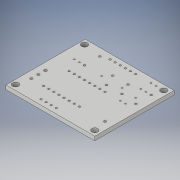
# Autodesk Inventor part: bard
Saved by Autodesk Inventor 2019 (Build 230136000, 136)
## iProperties
Created: 2020-01-03
Part Number: bard
Material: Типовые
Document SubType Name: Modeling
Designer: Петров Иван
Density: 1 g/cm^3
Appearance: По умолчанию
Author: Петров Иван
Autodesk Inventor part; units mm, degrees
ref_plane "YZ Plane" through (0, 0, 0) normal (1, 0, 0) x (0, 1, 0)
ref_plane "XZ Plane" through (0, 0, 0) normal (0, 1, 0) x (-1, 0, 0)
ref_plane "XY Plane" through (0, 0, 0) normal (0, 0, 1) x (1, 0, 0)
sketch "Эскиз1" plane through (0, 0, 0) normal (0, 1, 0) x (-1, 0, 0)
  arc A0 (18.669, 20.0698) -> (19.177, 20.0622) centre (18.923, 20.066) ccw
  arc A1 (19.304, 28.4442) -> (18.796, 28.4518) centre (19.05, 28.448) ccw
  line L0 (18.923, 20.066) -> (19.05, 28.448)
  arc A2 (32.004, 28.575) -> (31.496, 28.575) centre (31.75, 28.575) ccw
  line L1 (31.75, 28.575) -> (31.75, 21.209)
  arc A3 (31.496, 21.209) -> (32.004, 21.209) centre (31.75, 21.209) ccw
  arc A4 (34.163, 20.0622) -> (34.671, 20.0698) centre (34.417, 20.066) ccw
  arc A5 (34.544, 28.5788) -> (34.036, 28.5712) centre (34.29, 28.575) ccw
  line L2 (34.29, 28.575) -> (34.417, 20.066)
  line L3 (0, 0) -> (44.12, 0)
  line L4 (44.12, 0) -> (44.12, 39.36)
  line L5 (44.12, 39.36) -> (0, 39.36)
  line L6 (0, 39.36) -> (0, 0)
  circle A6 centre (2.54, 36.83) radius 1.5
  circle A7 centre (41.91, 36.83) radius 1.5
  circle A8 centre (41.91, 2.54) radius 1.5
  circle A9 centre (2.54, 2.54) radius 1.5
  line L7 (15.24, 5.588) -> (15.24, 0)
  arc A10 (16.51, 0.0318) -> (16.51, -0.0318) centre (16.51, 0) ccw
  line L8 (30.48, 5.588) -> (30.48, 0)
  arc A11 (30.4482, 0) -> (30.5118, 0) centre (30.48, 0) ccw
  arc A12 (30.5118, 5.588) -> (30.4482, 5.588) centre (30.48, 5.588) ccw
  arc A13 (15.24, 5.6197) -> (15.24, 5.5563) centre (15.24, 5.588) ccw
  arc A14 (15.2082, 0) -> (15.2718, 0) centre (15.24, 0) ccw
  arc A15 (15.2718, 5.588) -> (15.2082, 5.588) centre (15.24, 5.588) ccw
  line L9 (15.24, 5.588) -> (30.48, 5.588)
  arc A16 (30.48, 5.5563) -> (30.48, 5.6197) centre (30.48, 5.588) ccw
  arc A17 (29.21, -0.0318) -> (29.21, 0.0318) centre (29.21, 0) ccw
  line L10 (15.24, 0) -> (16.51, 0)
  arc A18 (16.51, -0.0318) -> (16.51, 0.0318) centre (16.51, 0) ccw
  arc A19 (15.24, 0.0318) -> (15.24, -0.0318) centre (15.24, 0) ccw
  line L11 (16.51, 0) -> (29.21, 0)
  arc A20 (16.51, 1.3017) -> (16.51, 1.2383) centre (16.51, 1.27) ccw
  arc A21 (29.21, 1.2383) -> (29.21, 1.3017) centre (29.21, 1.27) ccw
  line L12 (16.51, 1.27) -> (16.51, 0)
  arc A22 (16.4783, 0) -> (16.5418, 0) centre (16.5101, 0) ccw
  arc A23 (16.5418, 1.27) -> (16.4783, 1.27) centre (16.5101, 1.27) ccw
  line L13 (29.845, 3.81) -> (28.575, 3.81)
  arc A24 (28.575, 3.8608) -> (28.575, 3.7592) centre (28.575, 3.81) ccw
  arc A25 (29.845, 3.7592) -> (29.845, 3.8608) centre (29.845, 3.81) ccw
  arc A26 (29.1783, 0) -> (29.2418, 0) centre (29.2101, 0) ccw
  arc A27 (29.21, 0.0318) -> (29.21, -0.0318) centre (29.21, 0) ccw
  arc A28 (29.2418, 1.27) -> (29.1783, 1.27) centre (29.2101, 1.27) ccw
  line L14 (29.21, 1.27) -> (16.51, 1.27)
  line L15 (29.21, 0) -> (29.21, 1.27)
  arc A29 (30.48, -0.0318) -> (30.48, 0.0318) centre (30.48, 0) ccw
  line L16 (29.21, 0) -> (30.48, 0)
  line L17 (30.1498, 37.7698) -> (28.2702, 37.7698)
  line L18 (28.2702, 37.7698) -> (28.2702, 35.8902)
  line L19 (28.2702, 35.8902) -> (30.1498, 35.8902)
  line L20 (30.1498, 35.8902) -> (30.1498, 37.7698)
  line L21 (30.1498, 37.7698) -> (28.2702, 37.7698)
  line L22 (28.2702, 37.7698) -> (28.2702, 35.8902)
  line L23 (28.2702, 35.8902) -> (30.1498, 35.8902)
  line L24 (30.1498, 35.8902) -> (30.1498, 37.7698)
  arc A30 (26.67, 37.2999) -> (26.67, 36.3601) centre (26.67, 36.83) ccw
  arc A31 (26.67, 36.3601) -> (26.67, 37.2999) centre (26.67, 36.83) ccw
  arc A32 (26.67, 37.2999) -> (26.67, 36.3601) centre (26.67, 36.83) ccw
  arc A33 (26.67, 36.3601) -> (26.67, 37.2999) centre (26.67, 36.83) ccw
  arc A34 (24.13, 37.2999) -> (24.13, 36.3601) centre (24.13, 36.83) ccw
  arc A35 (24.13, 36.3601) -> (24.13, 37.2999) centre (24.13, 36.83) ccw
  arc A36 (24.13, 37.2999) -> (24.13, 36.3601) centre (24.13, 36.83) ccw
  arc A37 (24.13, 36.3601) -> (24.13, 37.2999) centre (24.13, 36.83) ccw
  arc A38 (21.59, 37.2999) -> (21.59, 36.3601) centre (21.59, 36.83) ccw
  arc A39 (21.59, 36.3601) -> (21.59, 37.2999) centre (21.59, 36.83) ccw
  arc A40 (21.59, 37.2999) -> (21.59, 36.3601) centre (21.59, 36.83) ccw
  arc A41 (21.59, 36.3601) -> (21.59, 37.2999) centre (21.59, 36.83) ccw
  arc A42 (29.21, 3.0099) -> (29.21, 2.0701) centre (29.21, 2.54) ccw
  arc A43 (29.21, 2.0701) -> (29.21, 3.0099) centre (29.21, 2.54) ccw
  arc A44 (29.21, 3.0099) -> (29.21, 2.0701) centre (29.21, 2.54) ccw
  arc A45 (29.21, 2.0701) -> (29.21, 3.0099) centre (29.21, 2.54) ccw
  arc A46 (26.67, 3.0099) -> (26.67, 2.0701) centre (26.67, 2.54) ccw
  arc A47 (26.67, 2.0701) -> (26.67, 3.0099) centre (26.67, 2.54) ccw
  arc A48 (26.67, 3.0099) -> (26.67, 2.0701) centre (26.67, 2.54) ccw
  arc A49 (26.67, 2.0701) -> (26.67, 3.0099) centre (26.67, 2.54) ccw
  arc A50 (24.13, 3.0099) -> (24.13, 2.0701) centre (24.13, 2.54) ccw
  arc A51 (24.13, 2.0701) -> (24.13, 3.0099) centre (24.13, 2.54) ccw
  arc A52 (24.13, 3.0099) -> (24.13, 2.0701) centre (24.13, 2.54) ccw
  arc A53 (24.13, 2.0701) -> (24.13, 3.0099) centre (24.13, 2.54) ccw
  arc A54 (21.59, 3.0099) -> (21.59, 2.0701) centre (21.59, 2.54) ccw
  arc A55 (21.59, 2.0701) -> (21.59, 3.0099) centre (21.59, 2.54) ccw
  arc A56 (21.59, 3.0099) -> (21.59, 2.0701) centre (21.59, 2.54) ccw
  arc A57 (21.59, 2.0701) -> (21.59, 3.0099) centre (21.59, 2.54) ccw
  arc A58 (19.05, 3.0099) -> (19.05, 2.0701) centre (19.05, 2.54) ccw
  arc A59 (19.05, 2.0701) -> (19.05, 3.0099) centre (19.05, 2.54) ccw
  arc A60 (19.05, 3.0099) -> (19.05, 2.0701) centre (19.05, 2.54) ccw
  arc A61 (19.05, 2.0701) -> (19.05, 3.0099) centre (19.05, 2.54) ccw
  arc A62 (16.51, 3.0099) -> (16.51, 2.0701) centre (16.51, 2.54) ccw
  arc A63 (16.51, 2.0701) -> (16.51, 3.0099) centre (16.51, 2.54) ccw
  arc A64 (16.51, 3.0099) -> (16.51, 2.0701) centre (16.51, 2.54) ccw
  arc A65 (16.51, 2.0701) -> (16.51, 3.0099) centre (16.51, 2.54) ccw
  line L25 (41.7195, 22.1455) -> (41.7195, 24.5585)
  line L26 (41.7195, 24.5585) -> (39.3065, 24.5585)
  line L27 (39.3065, 24.5585) -> (39.3065, 22.1455)
  line L28 (39.3065, 22.1455) -> (41.7195, 22.1455)
  line L29 (41.7195, 22.1455) -> (41.7195, 24.5585)
  line L30 (41.7195, 24.5585) -> (39.3065, 24.5585)
  line L31 (39.3065, 24.5585) -> (39.3065, 22.1455)
  line L32 (39.3065, 22.1455) -> (41.7195, 22.1455)
  arc A66 (41.1163, 26.852) -> (39.9098, 26.852) centre (40.513, 26.852) ccw
  arc A67 (39.9098, 26.852) -> (41.1163, 26.852) centre (40.513, 26.852) ccw
  arc A68 (41.1163, 26.852) -> (39.9098, 26.852) centre (40.513, 26.852) ccw
  arc A69 (39.9098, 26.852) -> (41.1163, 26.852) centre (40.513, 26.852) ccw
  arc A70 (41.1163, 30.352) -> (39.9098, 30.352) centre (40.513, 30.352) ccw
  arc A71 (39.9098, 30.352) -> (41.1163, 30.352) centre (40.513, 30.352) ccw
  arc A72 (41.1163, 30.352) -> (39.9098, 30.352) centre (40.513, 30.352) ccw
  arc A73 (39.9098, 30.352) -> (41.1163, 30.352) centre (40.513, 30.352) ccw
  line L33 (2.6035, 31.6865) -> (2.6035, 29.2735)
  line L34 (2.6035, 29.2735) -> (5.0165, 29.2735)
  line L35 (5.0165, 29.2735) -> (5.0165, 31.6865)
  line L36 (5.0165, 31.6865) -> (2.6035, 31.6865)
  line L37 (2.6035, 31.6865) -> (2.6035, 29.2735)
  line L38 (2.6035, 29.2735) -> (5.0165, 29.2735)
  line L39 (5.0165, 29.2735) -> (5.0165, 31.6865)
  line L40 (5.0165, 31.6865) -> (2.6035, 31.6865)
  arc A74 (3.2067, 26.98) -> (4.4133, 26.98) centre (3.81, 26.98) ccw
  arc A75 (4.4133, 26.98) -> (3.2068, 26.98) centre (3.81, 26.98) ccw
  arc A76 (3.2067, 26.98) -> (4.4133, 26.98) centre (3.81, 26.98) ccw
  arc A77 (4.4133, 26.98) -> (3.2068, 26.98) centre (3.81, 26.98) ccw
  arc A78 (3.2068, 23.48) -> (4.4132, 23.48) centre (3.81, 23.48) ccw
  arc A79 (4.4133, 23.48) -> (3.2068, 23.48) centre (3.81, 23.48) ccw
  arc A80 (3.2068, 23.48) -> (4.4132, 23.48) centre (3.81, 23.48) ccw
  arc A81 (4.4133, 23.48) -> (3.2068, 23.48) centre (3.81, 23.48) ccw
  line L41 (9.2202, 12.8368) -> (9.2202, 12.5632)
  line L42 (9.2202, 12.5632) -> (9.0268, 12.3698)
  line L43 (9.0268, 12.3698) -> (8.7532, 12.3698)
  line L44 (8.7532, 12.3698) -> (8.5598, 12.5632)
  line L45 (8.5598, 12.5632) -> (8.5598, 12.8368)
  line L46 (8.5598, 12.8368) -> (8.7532, 13.0302)
  line L47 (8.7532, 13.0302) -> (9.0268, 13.0302)
  line L48 (9.0268, 13.0302) -> (9.2202, 12.8368)
  line L49 (9.2202, 12.8368) -> (9.2202, 12.5632)
  line L50 (9.2202, 12.8368) -> (9.2202, 12.5632)
  line L51 (9.2202, 12.5632) -> (9.0268, 12.3698)
  line L52 (9.0268, 12.3698) -> (8.7532, 12.3698)
  line L53 (8.7532, 12.3698) -> (8.5598, 12.5632)
  line L54 (8.5598, 12.5632) -> (8.5598, 12.8368)
  line L55 (8.5598, 12.8368) -> (8.7532, 13.0302)
  line L56 (8.7532, 13.0302) -> (9.0268, 13.0302)
  line L57 (9.0268, 13.0302) -> (9.2202, 12.8368)
  line L58 (9.2202, 12.8368) -> (9.2202, 12.5632)
  line L59 (6.6802, 12.8368) -> (6.6802, 12.5632)
  line L60 (6.6802, 12.5632) -> (6.4868, 12.3698)
  line L61 (6.4868, 12.3698) -> (6.2132, 12.3698)
  line L62 (6.2132, 12.3698) -> (6.0198, 12.5632)
  line L63 (6.0198, 12.5632) -> (6.0198, 12.8368)
  line L64 (6.0198, 12.8368) -> (6.2132, 13.0302)
  line L65 (6.2132, 13.0302) -> (6.4868, 13.0302)
  line L66 (6.4868, 13.0302) -> (6.6802, 12.8368)
  line L67 (6.6802, 12.8368) -> (6.6802, 12.5632)
  line L68 (6.6802, 12.8368) -> (6.6802, 12.5632)
  line L69 (6.6802, 12.5632) -> (6.4868, 12.3698)
  line L70 (6.4868, 12.3698) -> (6.2132, 12.3698)
  line L71 (6.2132, 12.3698) -> (6.0198, 12.5632)
  line L72 (6.0198, 12.5632) -> (6.0198, 12.8368)
  line L73 (6.0198, 12.8368) -> (6.2132, 13.0302)
  line L74 (6.2132, 13.0302) -> (6.4868, 13.0302)
  line L75 (6.4868, 13.0302) -> (6.6802, 12.8368)
  line L76 (6.6802, 12.8368) -> (6.6802, 12.5632)
  line L77 (9.2202, 7.7568) -> (9.2202, 7.4832)
  line L78 (9.2202, 7.4832) -> (9.0268, 7.2898)
  line L79 (9.0268, 7.2898) -> (8.7532, 7.2898)
  line L80 (8.7532, 7.2898) -> (8.5598, 7.4832)
  line L81 (8.5598, 7.4832) -> (8.5598, 7.7568)
  line L82 (8.5598, 7.7568) -> (8.7532, 7.9502)
  line L83 (8.7532, 7.9502) -> (9.0268, 7.9502)
  line L84 (9.0268, 7.9502) -> (9.2202, 7.7568)
  line L85 (9.2202, 7.7568) -> (9.2202, 7.4832)
  line L86 (9.2202, 7.7568) -> (9.2202, 7.4832)
  line L87 (9.2202, 7.4832) -> (9.0268, 7.2898)
  line L88 (9.0268, 7.2898) -> (8.7532, 7.2898)
  line L89 (8.7532, 7.2898) -> (8.5598, 7.4832)
  line L90 (8.5598, 7.4832) -> (8.5598, 7.7568)
  line L91 (8.5598, 7.7568) -> (8.7532, 7.9502)
  line L92 (8.7532, 7.9502) -> (9.0268, 7.9502)
  line L93 (9.0268, 7.9502) -> (9.2202, 7.7568)
  line L94 (9.2202, 7.7568) -> (9.2202, 7.4832)
  line L95 (6.6802, 7.7568) -> (6.6802, 7.4832)
  line L96 (6.6802, 7.4832) -> (6.4868, 7.2898)
  line L97 (6.4868, 7.2898) -> (6.2132, 7.2898)
  line L98 (6.2132, 7.2898) -> (6.0198, 7.4832)
  line L99 (6.0198, 7.4832) -> (6.0198, 7.7568)
  line L100 (6.0198, 7.7568) -> (6.2132, 7.9502)
  line L101 (6.2132, 7.9502) -> (6.4868, 7.9502)
  line L102 (6.4868, 7.9502) -> (6.6802, 7.7568)
  line L103 (6.6802, 7.7568) -> (6.6802, 7.4832)
  line L104 (6.6802, 7.7568) -> (6.6802, 7.4832)
  line L105 (6.6802, 7.4832) -> (6.4868, 7.2898)
  line L106 (6.4868, 7.2898) -> (6.2132, 7.2898)
  line L107 (6.2132, 7.2898) -> (6.0198, 7.4832)
  line L108 (6.0198, 7.4832) -> (6.0198, 7.7568)
  line L109 (6.0198, 7.7568) -> (6.2132, 7.9502)
  line L110 (6.2132, 7.9502) -> (6.4868, 7.9502)
  line L111 (6.4868, 7.9502) -> (6.6802, 7.7568)
  line L112 (6.6802, 7.7568) -> (6.6802, 7.4832)
  line L113 (9.2202, 17.9168) -> (9.2202, 17.6432)
  line L114 (9.2202, 17.6432) -> (9.0268, 17.4498)
  line L115 (9.0268, 17.4498) -> (8.7532, 17.4498)
  line L116 (8.7532, 17.4498) -> (8.5598, 17.6432)
  line L117 (8.5598, 17.6432) -> (8.5598, 17.9168)
  line L118 (8.5598, 17.9168) -> (8.7532, 18.1102)
  line L119 (8.7532, 18.1102) -> (9.0268, 18.1102)
  line L120 (9.0268, 18.1102) -> (9.2202, 17.9168)
  line L121 (9.2202, 17.9168) -> (9.2202, 17.6432)
  line L122 (9.2202, 17.9168) -> (9.2202, 17.6432)
  line L123 (9.2202, 17.6432) -> (9.0268, 17.4498)
  line L124 (9.0268, 17.4498) -> (8.7532, 17.4498)
  line L125 (8.7532, 17.4498) -> (8.5598, 17.6432)
  line L126 (8.5598, 17.6432) -> (8.5598, 17.9168)
  line L127 (8.5598, 17.9168) -> (8.7532, 18.1102)
  line L128 (8.7532, 18.1102) -> (9.0268, 18.1102)
  line L129 (9.0268, 18.1102) -> (9.2202, 17.9168)
  line L130 (9.2202, 17.9168) -> (9.2202, 17.6432)
  line L131 (6.6802, 17.9168) -> (6.6802, 17.6432)
  line L132 (6.6802, 17.6432) -> (6.4868, 17.4498)
  line L133 (6.4868, 17.4498) -> (6.2132, 17.4498)
  line L134 (6.2132, 17.4498) -> (6.0198, 17.6432)
  line L135 (6.0198, 17.6432) -> (6.0198, 17.9168)
  line L136 (6.0198, 17.9168) -> (6.2132, 18.1102)
  line L137 (6.2132, 18.1102) -> (6.4868, 18.1102)
  line L138 (6.4868, 18.1102) -> (6.6802, 17.9168)
  line L139 (6.6802, 17.9168) -> (6.6802, 17.6432)
  line L140 (6.6802, 17.9168) -> (6.6802, 17.6432)
  line L141 (6.6802, 17.6432) -> (6.4868, 17.4498)
  line L142 (6.4868, 17.4498) -> (6.2132, 17.4498)
  line L143 (6.2132, 17.4498) -> (6.0198, 17.6432)
  line L144 (6.0198, 17.6432) -> (6.0198, 17.9168)
  line L145 (6.0198, 17.9168) -> (6.2132, 18.1102)
  line L146 (6.2132, 18.1102) -> (6.4868, 18.1102)
  line L147 (6.4868, 18.1102) -> (6.6802, 17.9168)
  line L148 (6.6802, 17.9168) -> (6.6802, 17.6432)
  line L149 (35.2298, 11.2932) -> (35.2298, 11.5668)
  line L150 (35.2298, 11.5668) -> (35.4232, 11.7602)
  line L151 (35.4232, 11.7602) -> (35.6968, 11.7602)
  line L152 (35.6968, 11.7602) -> (35.8902, 11.5668)
  line L153 (35.8902, 11.5668) -> (35.8902, 11.2932)
  line L154 (35.8902, 11.2932) -> (35.6968, 11.0998)
  line L155 (35.6968, 11.0998) -> (35.4232, 11.0998)
  line L156 (35.4232, 11.0998) -> (35.2298, 11.2932)
  line L157 (35.2298, 11.2932) -> (35.2298, 11.5668)
  line L158 (35.2298, 11.2932) -> (35.2298, 11.5668)
  line L159 (35.2298, 11.5668) -> (35.4232, 11.7602)
  line L160 (35.4232, 11.7602) -> (35.6968, 11.7602)
  line L161 (35.6968, 11.7602) -> (35.8902, 11.5668)
  line L162 (35.8902, 11.5668) -> (35.8902, 11.2932)
  line L163 (35.8902, 11.2932) -> (35.6968, 11.0998)
  line L164 (35.6968, 11.0998) -> (35.4232, 11.0998)
  line L165 (35.4232, 11.0998) -> (35.2298, 11.2932)
  line L166 (35.2298, 11.2932) -> (35.2298, 11.5668)
  line L167 (37.7698, 11.2932) -> (37.7698, 11.5668)
  line L168 (37.7698, 11.5668) -> (37.9632, 11.7602)
  line L169 (37.9632, 11.7602) -> (38.2368, 11.7602)
  line L170 (38.2368, 11.7602) -> (38.4302, 11.5668)
  line L171 (38.4302, 11.5668) -> (38.4302, 11.2932)
  line L172 (38.4302, 11.2932) -> (38.2368, 11.0998)
  line L173 (38.2368, 11.0998) -> (37.9632, 11.0998)
  line L174 (37.9632, 11.0998) -> (37.7698, 11.2932)
  line L175 (37.7698, 11.2932) -> (37.7698, 11.5668)
  line L176 (37.7698, 11.2932) -> (37.7698, 11.5668)
  line L177 (37.7698, 11.5668) -> (37.9632, 11.7602)
  line L178 (37.9632, 11.7602) -> (38.2368, 11.7602)
  line L179 (38.2368, 11.7602) -> (38.4302, 11.5668)
  line L180 (38.4302, 11.5668) -> (38.4302, 11.2932)
  line L181 (38.4302, 11.2932) -> (38.2368, 11.0998)
  line L182 (38.2368, 11.0998) -> (37.9632, 11.0998)
  line L183 (37.9632, 11.0998) -> (37.7698, 11.2932)
  line L184 (37.7698, 11.2932) -> (37.7698, 11.5668)
  line L185 (6.0198, 2.4032) -> (6.0198, 2.6768)
  line L186 (6.0198, 2.6768) -> (6.2132, 2.8702)
  line L187 (6.2132, 2.8702) -> (6.4868, 2.8702)
  line L188 (6.4868, 2.8702) -> (6.6802, 2.6768)
  line L189 (6.6802, 2.6768) -> (6.6802, 2.4032)
  line L190 (6.6802, 2.4032) -> (6.4868, 2.2098)
  line L191 (6.4868, 2.2098) -> (6.2132, 2.2098)
  line L192 (6.2132, 2.2098) -> (6.0198, 2.4032)
  line L193 (6.0198, 2.4032) -> (6.0198, 2.6768)
  line L194 (6.0198, 2.4032) -> (6.0198, 2.6768)
  line L195 (6.0198, 2.6768) -> (6.2132, 2.8702)
  line L196 (6.2132, 2.8702) -> (6.4868, 2.8702)
  line L197 (6.4868, 2.8702) -> (6.6802, 2.6768)
  line L198 (6.6802, 2.6768) -> (6.6802, 2.4032)
  line L199 (6.6802, 2.4032) -> (6.4868, 2.2098)
  line L200 (6.4868, 2.2098) -> (6.2132, 2.2098)
  line L201 (6.2132, 2.2098) -> (6.0198, 2.4032)
  line L202 (6.0198, 2.4032) -> (6.0198, 2.6768)
  line L203 (8.5598, 2.4032) -> (8.5598, 2.6768)
  line L204 (8.5598, 2.6768) -> (8.7532, 2.8702)
  line L205 (8.7532, 2.8702) -> (9.0268, 2.8702)
  line L206 (9.0268, 2.8702) -> (9.2202, 2.6768)
  line L207 (9.2202, 2.6768) -> (9.2202, 2.4032)
  line L208 (9.2202, 2.4032) -> (9.0268, 2.2098)
  line L209 (9.0268, 2.2098) -> (8.7532, 2.2098)
  line L210 (8.7532, 2.2098) -> (8.5598, 2.4032)
  line L211 (8.5598, 2.4032) -> (8.5598, 2.6768)
  line L212 (8.5598, 2.4032) -> (8.5598, 2.6768)
  line L213 (8.5598, 2.6768) -> (8.7532, 2.8702)
  line L214 (8.7532, 2.8702) -> (9.0268, 2.8702)
  line L215 (9.0268, 2.8702) -> (9.2202, 2.6768)
  line L216 (9.2202, 2.6768) -> (9.2202, 2.4032)
  line L217 (9.2202, 2.4032) -> (9.0268, 2.2098)
  line L218 (9.0268, 2.2098) -> (8.7532, 2.2098)
  line L219 (8.7532, 2.2098) -> (8.5598, 2.4032)
  line L220 (8.5598, 2.4032) -> (8.5598, 2.6768)
  line L221 (13.6398, 11.6742) -> (13.6398, 11.9478)
  line L222 (13.6398, 11.9478) -> (13.8332, 12.1412)
  line L223 (13.8332, 12.1412) -> (14.1068, 12.1412)
  line L224 (14.1068, 12.1412) -> (14.3002, 11.9478)
  line L225 (14.3002, 11.9478) -> (14.3002, 11.6742)
  line L226 (14.3002, 11.6742) -> (14.1068, 11.4808)
  line L227 (14.1068, 11.4808) -> (13.8332, 11.4808)
  line L228 (13.8332, 11.4808) -> (13.6398, 11.6742)
  line L229 (13.6398, 11.6742) -> (13.6398, 11.9478)
  line L230 (13.6398, 11.6742) -> (13.6398, 11.9478)
  line L231 (13.6398, 11.9478) -> (13.8332, 12.1412)
  line L232 (13.8332, 12.1412) -> (14.1068, 12.1412)
  line L233 (14.1068, 12.1412) -> (14.3002, 11.9478)
  line L234 (14.3002, 11.9478) -> (14.3002, 11.6742)
  line L235 (14.3002, 11.6742) -> (14.1068, 11.4808)
  line L236 (14.1068, 11.4808) -> (13.8332, 11.4808)
  line L237 (13.8332, 11.4808) -> (13.6398, 11.6742)
  line L238 (13.6398, 11.6742) -> (13.6398, 11.9478)
  line L239 (23.7998, 11.6742) -> (23.7998, 11.9478)
  line L240 (23.7998, 11.9478) -> (23.9932, 12.1412)
  line L241 (23.9932, 12.1412) -> (24.2668, 12.1412)
  line L242 (24.2668, 12.1412) -> (24.4602, 11.9478)
  line L243 (24.4602, 11.9478) -> (24.4602, 11.6742)
  line L244 (24.4602, 11.6742) -> (24.2668, 11.4808)
  line L245 (24.2668, 11.4808) -> (23.9932, 11.4808)
  line L246 (23.9932, 11.4808) -> (23.7998, 11.6742)
  line L247 (23.7998, 11.6742) -> (23.7998, 11.9478)
  line L248 (23.7998, 11.6742) -> (23.7998, 11.9478)
  line L249 (23.7998, 11.9478) -> (23.9932, 12.1412)
  line L250 (23.9932, 12.1412) -> (24.2668, 12.1412)
  line L251 (24.2668, 12.1412) -> (24.4602, 11.9478)
  line L252 (24.4602, 11.9478) -> (24.4602, 11.6742)
  line L253 (24.4602, 11.6742) -> (24.2668, 11.4808)
  line L254 (24.2668, 11.4808) -> (23.9932, 11.4808)
  line L255 (23.9932, 11.4808) -> (23.7998, 11.6742)
  line L256 (23.7998, 11.6742) -> (23.7998, 11.9478)
  line L257 (13.4874, 8.69) -> (13.4874, 9.09)
  line L258 (13.4874, 9.09) -> (13.77, 9.3726)
  line L259 (13.77, 9.3726) -> (14.17, 9.3726)
  line L260 (14.17, 9.3726) -> (14.4526, 9.09)
  line L261 (14.4526, 9.09) -> (14.4526, 8.69)
  line L262 (14.4526, 8.69) -> (14.17, 8.4074)
  line L263 (14.17, 8.4074) -> (13.77, 8.4074)
  line L264 (13.77, 8.4074) -> (13.4874, 8.69)
  line L265 (13.4874, 8.69) -> (13.4874, 9.09)
  line L266 (13.4874, 8.69) -> (13.4874, 9.09)
  line L267 (13.4874, 9.09) -> (13.77, 9.3726)
  line L268 (13.77, 9.3726) -> (14.17, 9.3726)
  line L269 (14.17, 9.3726) -> (14.4526, 9.09)
  line L270 (14.4526, 9.09) -> (14.4526, 8.69)
  line L271 (14.4526, 8.69) -> (14.17, 8.4074)
  line L272 (14.17, 8.4074) -> (13.77, 8.4074)
  line L273 (13.77, 8.4074) -> (13.4874, 8.69)
  line L274 (13.4874, 8.69) -> (13.4874, 9.09)
  line L275 (21.1074, 8.69) -> (21.1074, 9.09)
  line L276 (21.1074, 9.09) -> (21.39, 9.3726)
  line L277 (21.39, 9.3726) -> (21.79, 9.3726)
  line L278 (21.79, 9.3726) -> (22.0726, 9.09)
  line L279 (22.0726, 9.09) -> (22.0726, 8.69)
  line L280 (22.0726, 8.69) -> (21.79, 8.4074)
  line L281 (21.79, 8.4074) -> (21.39, 8.4074)
  line L282 (21.39, 8.4074) -> (21.1074, 8.69)
  line L283 (21.1074, 8.69) -> (21.1074, 9.09)
  line L284 (21.1074, 8.69) -> (21.1074, 9.09)
  line L285 (21.1074, 9.09) -> (21.39, 9.3726)
  line L286 (21.39, 9.3726) -> (21.79, 9.3726)
  line L287 (21.79, 9.3726) -> (22.0726, 9.09)
  line L288 (22.0726, 9.09) -> (22.0726, 8.69)
  line L289 (22.0726, 8.69) -> (21.79, 8.4074)
  line L290 (21.79, 8.4074) -> (21.39, 8.4074)
  line L291 (21.39, 8.4074) -> (21.1074, 8.69)
  line L292 (21.1074, 8.69) -> (21.1074, 9.09)
  line L293 (10.9474, 14.278) -> (10.9474, 14.678)
  line L294 (10.9474, 14.678) -> (11.23, 14.9606)
  line L295 (11.23, 14.9606) -> (11.63, 14.9606)
  line L296 (11.63, 14.9606) -> (11.9126, 14.678)
  line L297 (11.9126, 14.678) -> (11.9126, 14.278)
  line L298 (11.9126, 14.278) -> (11.63, 13.9954)
  line L299 (11.63, 13.9954) -> (11.23, 13.9954)
  line L300 (11.23, 13.9954) -> (10.9474, 14.278)
  line L301 (10.9474, 14.278) -> (10.9474, 14.678)
  line L302 (10.9474, 14.278) -> (10.9474, 14.678)
  line L303 (10.9474, 14.678) -> (11.23, 14.9606)
  line L304 (11.23, 14.9606) -> (11.63, 14.9606)
  line L305 (11.63, 14.9606) -> (11.9126, 14.678)
  line L306 (11.9126, 14.678) -> (11.9126, 14.278)
  line L307 (11.9126, 14.278) -> (11.63, 13.9954)
  line L308 (11.63, 13.9954) -> (11.23, 13.9954)
  line L309 (11.23, 13.9954) -> (10.9474, 14.278)
  line L310 (10.9474, 14.278) -> (10.9474, 14.678)
  line L311 (18.5674, 14.278) -> (18.5674, 14.678)
  line L312 (18.5674, 14.678) -> (18.85, 14.9606)
  line L313 (18.85, 14.9606) -> (19.25, 14.9606)
  line L314 (19.25, 14.9606) -> (19.5326, 14.678)
  line L315 (19.5326, 14.678) -> (19.5326, 14.278)
  line L316 (19.5326, 14.278) -> (19.25, 13.9954)
  line L317 (19.25, 13.9954) -> (18.85, 13.9954)
  line L318 (18.85, 13.9954) -> (18.5674, 14.278)
  line L319 (18.5674, 14.278) -> (18.5674, 14.678)
  line L320 (18.5674, 14.278) -> (18.5674, 14.678)
  line L321 (18.5674, 14.678) -> (18.85, 14.9606)
  line L322 (18.85, 14.9606) -> (19.25, 14.9606)
  line L323 (19.25, 14.9606) -> (19.5326, 14.678)
  line L324 (19.5326, 14.678) -> (19.5326, 14.278)
  line L325 (19.5326, 14.278) -> (19.25, 13.9954)
  line L326 (19.25, 13.9954) -> (18.85, 13.9954)
  line L327 (18.85, 13.9954) -> (18.5674, 14.278)
  line L328 (18.5674, 14.278) -> (18.5674, 14.678)
  line L329 (32.82, 11.9126) -> (33.22, 11.9126)
  line L330 (33.22, 11.9126) -> (33.5026, 11.63)
  line L331 (33.5026, 11.63) -> (33.5026, 11.23)
  line L332 (33.5026, 11.23) -> (33.22, 10.9474)
  line L333 (33.22, 10.9474) -> (32.82, 10.9474)
  line L334 (32.82, 10.9474) -> (32.5374, 11.23)
  line L335 (32.5374, 11.23) -> (32.5374, 11.63)
  line L336 (32.5374, 11.63) -> (32.82, 11.9126)
  line L337 (32.82, 11.9126) -> (33.22, 11.9126)
  line L338 (32.82, 11.9126) -> (33.22, 11.9126)
  line L339 (33.22, 11.9126) -> (33.5026, 11.63)
  line L340 (33.5026, 11.63) -> (33.5026, 11.23)
  line L341 (33.5026, 11.23) -> (33.22, 10.9474)
  line L342 (33.22, 10.9474) -> (32.82, 10.9474)
  line L343 (32.82, 10.9474) -> (32.5374, 11.23)
  line L344 (32.5374, 11.23) -> (32.5374, 11.63)
  line L345 (32.5374, 11.63) -> (32.82, 11.9126)
  line L346 (32.82, 11.9126) -> (33.22, 11.9126)
  line L347 (32.82, 4.2926) -> (33.22, 4.2926)
  line L348 (33.22, 4.2926) -> (33.5026, 4.01)
  line L349 (33.5026, 4.01) -> (33.5026, 3.61)
  line L350 (33.5026, 3.61) -> (33.22, 3.3274)
  line L351 (33.22, 3.3274) -> (32.82, 3.3274)
  line L352 (32.82, 3.3274) -> (32.5374, 3.61)
  line L353 (32.5374, 3.61) -> (32.5374, 4.01)
  line L354 (32.5374, 4.01) -> (32.82, 4.2926)
  line L355 (32.82, 4.2926) -> (33.22, 4.2926)
  line L356 (32.82, 4.2926) -> (33.22, 4.2926)
  line L357 (33.22, 4.2926) -> (33.5026, 4.01)
  line L358 (33.5026, 4.01) -> (33.5026, 3.61)
  line L359 (33.5026, 3.61) -> (33.22, 3.3274)
  line L360 (33.22, 3.3274) -> (32.82, 3.3274)
  line L361 (32.82, 3.3274) -> (32.5374, 3.61)
  line L362 (32.5374, 3.61) -> (32.5374, 4.01)
  line L363 (32.5374, 4.01) -> (32.82, 4.2926)
  line L364 (32.82, 4.2926) -> (33.22, 4.2926)
  line L365 (3.883, 7.1374) -> (3.483, 7.1374)
  line L366 (3.483, 7.1374) -> (3.2004, 7.42)
  line L367 (3.2004, 7.42) -> (3.2004, 7.82)
  line L368 (3.2004, 7.82) -> (3.483, 8.1026)
  line L369 (3.483, 8.1026) -> (3.883, 8.1026)
  line L370 (3.883, 8.1026) -> (4.1656, 7.82)
  line L371 (4.1656, 7.82) -> (4.1656, 7.42)
  line L372 (4.1656, 7.42) -> (3.883, 7.1374)
  line L373 (3.883, 7.1374) -> (3.483, 7.1374)
  line L374 (3.883, 7.1374) -> (3.483, 7.1374)
  line L375 (3.483, 7.1374) -> (3.2004, 7.42)
  line L376 (3.2004, 7.42) -> (3.2004, 7.82)
  line L377 (3.2004, 7.82) -> (3.483, 8.1026)
  line L378 (3.483, 8.1026) -> (3.883, 8.1026)
  line L379 (3.883, 8.1026) -> (4.1656, 7.82)
  line L380 (4.1656, 7.82) -> (4.1656, 7.42)
  line L381 (4.1656, 7.42) -> (3.883, 7.1374)
  line L382 (3.883, 7.1374) -> (3.483, 7.1374)
  line L383 (3.883, 14.7574) -> (3.483, 14.7574)
  line L384 (3.483, 14.7574) -> (3.2004, 15.04)
  line L385 (3.2004, 15.04) -> (3.2004, 15.44)
  line L386 (3.2004, 15.44) -> (3.483, 15.7226)
  line L387 (3.483, 15.7226) -> (3.883, 15.7226)
  line L388 (3.883, 15.7226) -> (4.1656, 15.44)
  line L389 (4.1656, 15.44) -> (4.1656, 15.04)
  line L390 (4.1656, 15.04) -> (3.883, 14.7574)
  line L391 (3.883, 14.7574) -> (3.483, 14.7574)
  line L392 (3.883, 14.7574) -> (3.483, 14.7574)
  line L393 (3.483, 14.7574) -> (3.2004, 15.04)
  line L394 (3.2004, 15.04) -> (3.2004, 15.44)
  line L395 (3.2004, 15.44) -> (3.483, 15.7226)
  line L396 (3.483, 15.7226) -> (3.883, 15.7226)
  line L397 (3.883, 15.7226) -> (4.1656, 15.44)
  line L398 (4.1656, 15.44) -> (4.1656, 15.04)
  line L399 (4.1656, 15.04) -> (3.883, 14.7574)
  line L400 (3.883, 14.7574) -> (3.483, 14.7574)
  line L401 (16.51, 17.126) -> (16.51, 18.434)
  arc A82 (16.837, 18.434) -> (16.183, 18.434) centre (16.51, 18.434) ccw
  arc A83 (16.183, 17.126) -> (16.837, 17.126) centre (16.51, 17.126) ccw
  line L402 (16.51, 17.126) -> (16.51, 18.434)
  arc A84 (16.837, 18.434) -> (16.183, 18.434) centre (16.51, 18.434) ccw
  arc A85 (16.183, 17.126) -> (16.837, 17.126) centre (16.51, 17.126) ccw
  line L403 (19.05, 17.126) -> (19.05, 18.434)
  arc A86 (19.377, 18.434) -> (18.723, 18.434) centre (19.05, 18.434) ccw
  arc A87 (18.723, 17.126) -> (19.377, 17.126) centre (19.05, 17.126) ccw
  line L404 (19.05, 17.126) -> (19.05, 18.434)
  arc A88 (19.377, 18.434) -> (18.723, 18.434) centre (19.05, 18.434) ccw
  arc A89 (18.723, 17.126) -> (19.377, 17.126) centre (19.05, 17.126) ccw
  line L405 (21.59, 17.126) -> (21.59, 18.434)
  arc A90 (21.917, 18.434) -> (21.263, 18.434) centre (21.59, 18.434) ccw
  arc A91 (21.263, 17.126) -> (21.917, 17.126) centre (21.59, 17.126) ccw
  line L406 (21.59, 17.126) -> (21.59, 18.434)
  arc A92 (21.917, 18.434) -> (21.263, 18.434) centre (21.59, 18.434) ccw
  arc A93 (21.263, 17.126) -> (21.917, 17.126) centre (21.59, 17.126) ccw
  line L407 (24.13, 17.126) -> (24.13, 18.434)
  arc A94 (24.457, 18.434) -> (23.803, 18.434) centre (24.13, 18.434) ccw
  arc A95 (23.803, 17.126) -> (24.457, 17.126) centre (24.13, 17.126) ccw
  line L408 (24.13, 17.126) -> (24.13, 18.434)
  arc A96 (24.457, 18.434) -> (23.803, 18.434) centre (24.13, 18.434) ccw
  arc A97 (23.803, 17.126) -> (24.457, 17.126) centre (24.13, 17.126) ccw
  line L409 (26.67, 17.126) -> (26.67, 18.434)
  arc A98 (26.997, 18.434) -> (26.343, 18.434) centre (26.67, 18.434) ccw
  arc A99 (26.343, 17.126) -> (26.997, 17.126) centre (26.67, 17.126) ccw
  line L410 (26.67, 17.126) -> (26.67, 18.434)
  arc A100 (26.997, 18.434) -> (26.343, 18.434) centre (26.67, 18.434) ccw
  arc A101 (26.343, 17.126) -> (26.997, 17.126) centre (26.67, 17.126) ccw
  line L411 (29.21, 17.126) -> (29.21, 18.434)
  arc A102 (29.537, 18.434) -> (28.883, 18.434) centre (29.21, 18.434) ccw
  arc A103 (28.883, 17.126) -> (29.537, 17.126) centre (29.21, 17.126) ccw
  line L412 (29.21, 17.126) -> (29.21, 18.434)
  arc A104 (29.537, 18.434) -> (28.883, 18.434) centre (29.21, 18.434) ccw
  arc A105 (28.883, 17.126) -> (29.537, 17.126) centre (29.21, 17.126) ccw
  line L413 (31.75, 17.126) -> (31.75, 18.434)
  arc A106 (32.077, 18.434) -> (31.423, 18.434) centre (31.75, 18.434) ccw
  arc A107 (31.423, 17.126) -> (32.077, 17.126) centre (31.75, 17.126) ccw
  line L414 (31.75, 17.126) -> (31.75, 18.434)
  arc A108 (32.077, 18.434) -> (31.423, 18.434) centre (31.75, 18.434) ccw
  arc A109 (31.423, 17.126) -> (32.077, 17.126) centre (31.75, 17.126) ccw
  line L415 (34.29, 17.126) -> (34.29, 18.434)
  arc A110 (34.617, 18.434) -> (33.963, 18.434) centre (34.29, 18.434) ccw
  arc A111 (33.963, 17.126) -> (34.617, 17.126) centre (34.29, 17.126) ccw
  line L416 (34.29, 17.126) -> (34.29, 18.434)
  arc A112 (34.617, 18.434) -> (33.963, 18.434) centre (34.29, 18.434) ccw
  arc A113 (33.963, 17.126) -> (34.617, 17.126) centre (34.29, 17.126) ccw
  arc A114 (34.617, 31.134) -> (33.963, 31.134) centre (34.29, 31.134) ccw
  arc A115 (33.963, 29.826) -> (34.617, 29.826) centre (34.29, 29.826) ccw
  arc A116 (34.617, 31.134) -> (33.963, 31.134) centre (34.29, 31.134) ccw
  arc A117 (33.963, 29.826) -> (34.617, 29.826) centre (34.29, 29.826) ccw
  line L417 (31.75, 29.826) -> (31.75, 31.134)
  arc A118 (32.077, 31.134) -> (31.423, 31.134) centre (31.75, 31.134) ccw
  arc A119 (31.423, 29.826) -> (32.077, 29.826) centre (31.75, 29.826) ccw
  line L418 (31.75, 29.826) -> (31.75, 31.134)
  arc A120 (32.077, 31.134) -> (31.423, 31.134) centre (31.75, 31.134) ccw
  arc A121 (31.423, 29.826) -> (32.077, 29.826) centre (31.75, 29.826) ccw
  line L419 (29.21, 29.826) -> (29.21, 31.134)
  arc A122 (29.537, 31.134) -> (28.883, 31.134) centre (29.21, 31.134) ccw
  arc A123 (28.883, 29.826) -> (29.537, 29.826) centre (29.21, 29.826) ccw
  line L420 (29.21, 29.826) -> (29.21, 31.134)
  arc A124 (29.537, 31.134) -> (28.883, 31.134) centre (29.21, 31.134) ccw
  arc A125 (28.883, 29.826) -> (29.537, 29.826) centre (29.21, 29.826) ccw
  line L421 (26.67, 29.826) -> (26.67, 31.134)
  arc A126 (26.997, 31.134) -> (26.343, 31.134) centre (26.67, 31.134) ccw
  arc A127 (26.343, 29.826) -> (26.997, 29.826) centre (26.67, 29.826) ccw
  line L422 (26.67, 29.826) -> (26.67, 31.134)
  arc A128 (26.997, 31.134) -> (26.343, 31.134) centre (26.67, 31.134) ccw
  arc A129 (26.343, 29.826) -> (26.997, 29.826) centre (26.67, 29.826) ccw
  line L423 (24.13, 29.826) -> (24.13, 31.134)
  arc A130 (24.457, 31.134) -> (23.803, 31.134) centre (24.13, 31.134) ccw
  arc A131 (23.803, 29.826) -> (24.457, 29.826) centre (24.13, 29.826) ccw
  line L424 (24.13, 29.826) -> (24.13, 31.134)
  arc A132 (24.457, 31.134) -> (23.803, 31.134) centre (24.13, 31.134) ccw
  arc A133 (23.803, 29.826) -> (24.457, 29.826) centre (24.13, 29.826) ccw
  line L425 (21.59, 29.826) -> (21.59, 31.134)
  arc A134 (21.917, 31.134) -> (21.263, 31.134) centre (21.59, 31.134) ccw
  arc A135 (21.263, 29.826) -> (21.917, 29.826) centre (21.59, 29.826) ccw
  line L426 (21.59, 29.826) -> (21.59, 31.134)
  arc A136 (21.917, 31.134) -> (21.263, 31.134) centre (21.59, 31.134) ccw
  arc A137 (21.263, 29.826) -> (21.917, 29.826) centre (21.59, 29.826) ccw
  line L427 (19.05, 29.826) -> (19.05, 31.134)
  arc A138 (19.377, 31.134) -> (18.723, 31.134) centre (19.05, 31.134) ccw
  arc A139 (18.723, 29.826) -> (19.377, 29.826) centre (19.05, 29.826) ccw
  line L428 (19.05, 29.826) -> (19.05, 31.134)
  arc A140 (19.377, 31.134) -> (18.723, 31.134) centre (19.05, 31.134) ccw
  arc A141 (18.723, 29.826) -> (19.377, 29.826) centre (19.05, 29.826) ccw
  line L429 (16.51, 29.826) -> (16.51, 31.134)
  arc A142 (16.837, 31.134) -> (16.183, 31.134) centre (16.51, 31.134) ccw
  arc A143 (16.183, 29.826) -> (16.837, 29.826) centre (16.51, 29.826) ccw
  line L430 (16.51, 29.826) -> (16.51, 31.134)
  arc A144 (16.837, 31.134) -> (16.183, 31.134) centre (16.51, 31.134) ccw
  arc A145 (16.183, 29.826) -> (16.837, 29.826) centre (16.51, 29.826) ccw
  arc A146 (31.75, 20.9074) -> (31.75, 21.5106) centre (31.75, 21.209) ccw
  arc A147 (31.75, 21.5106) -> (31.75, 20.9074) centre (31.75, 21.209) ccw
  arc A148 (31.75, 20.9074) -> (31.75, 21.5106) centre (31.75, 21.209) ccw
  arc A149 (31.75, 21.5106) -> (31.75, 20.9074) centre (31.75, 21.209) ccw
  arc A150 (31.75, 28.2734) -> (31.75, 28.8766) centre (31.75, 28.575) ccw
  arc A151 (31.75, 28.8766) -> (31.75, 28.2734) centre (31.75, 28.575) ccw
  arc A152 (31.75, 28.2734) -> (31.75, 28.8766) centre (31.75, 28.575) ccw
  arc A153 (31.75, 28.8766) -> (31.75, 28.2734) centre (31.75, 28.575) ccw
  arc A154 (18.923, 19.7644) -> (18.923, 20.3676) centre (18.923, 20.066) ccw
  arc A155 (18.923, 20.3676) -> (18.923, 19.7644) centre (18.923, 20.066) ccw
  arc A156 (18.923, 19.7644) -> (18.923, 20.3676) centre (18.923, 20.066) ccw
  arc A157 (18.923, 20.3676) -> (18.923, 19.7644) centre (18.923, 20.066) ccw
  arc A158 (34.417, 19.7644) -> (34.417, 20.3676) centre (34.417, 20.066) ccw
  arc A159 (34.417, 20.3676) -> (34.417, 19.7644) centre (34.417, 20.066) ccw
  arc A160 (34.417, 19.7644) -> (34.417, 20.3676) centre (34.417, 20.066) ccw
  arc A161 (34.417, 20.3676) -> (34.417, 19.7644) centre (34.417, 20.066) ccw
  arc A162 (19.05, 28.1464) -> (19.05, 28.7496) centre (19.05, 28.448) ccw
  arc A163 (19.05, 28.7496) -> (19.05, 28.1464) centre (19.05, 28.448) ccw
  arc A164 (19.05, 28.1464) -> (19.05, 28.7496) centre (19.05, 28.448) ccw
  arc A165 (19.05, 28.7496) -> (19.05, 28.1464) centre (19.05, 28.448) ccw
  arc A166 (34.29, 28.2734) -> (34.29, 28.8766) centre (34.29, 28.575) ccw
  arc A167 (34.29, 28.8766) -> (34.29, 28.2734) centre (34.29, 28.575) ccw
  arc A168 (34.29, 28.2734) -> (34.29, 28.8766) centre (34.29, 28.575) ccw
  arc A169 (34.29, 28.8766) -> (34.29, 28.2734) centre (34.29, 28.575) ccw
  line L431 (44.12, 39.36) -> (0, 39.36)
  line L432 (0, 39.36) -> (0, 0)
  line L433 (0, 0) -> (44.12, 0)
  line L434 (44.12, 0) -> (44.12, 39.36)
  circle A170 centre (29.21, 36.83) radius 0.4699
  circle A171 centre (26.67, 36.83) radius 0.4699
  circle A172 centre (24.13, 36.83) radius 0.4699
  circle A173 centre (21.59, 36.83) radius 0.47
  circle A174 centre (40.513, 30.352) radius 0.6033
  circle A175 centre (40.513, 26.852) radius 0.6033
  circle A176 centre (40.513, 23.352) radius 0.7179
  circle A177 centre (38.1, 11.43) radius 0.3574
  circle A178 centre (35.56, 11.43) radius 0.3574
  circle A179 centre (33.02, 11.43) radius 0.5224
  circle A180 centre (33.02, 3.81) radius 0.5224
  circle A181 centre (29.21, 2.54) radius 0.4699
  circle A182 centre (26.67, 2.54) radius 0.4699
  circle A183 centre (24.13, 2.54) radius 0.4699
  circle A184 centre (21.59, 2.54) radius 0.4699
  circle A185 centre (19.05, 2.54) radius 0.4699
  circle A186 centre (16.51, 2.54) radius 0.4699
  circle A187 centre (24.13, 11.811) radius 0.3574
  circle A188 centre (21.59, 8.89) radius 0.5224
  circle A189 centre (19.05, 14.478) radius 0.5224
  circle A190 centre (11.43, 14.478) radius 0.5224
  circle A191 centre (13.97, 11.811) radius 0.3574
  circle A192 centre (13.97, 8.89) radius 0.5224
  circle A193 centre (8.89, 7.62) radius 0.3574
  circle A194 centre (8.89, 2.54) radius 0.3574
  circle A195 centre (6.35, 2.54) radius 0.3574
  circle A196 centre (6.35, 7.62) radius 0.3574
  circle A197 centre (6.35, 12.7) radius 0.3574
  circle A198 centre (3.683, 7.62) radius 0.5224
  circle A199 centre (3.683, 15.24) radius 0.5224
  circle A200 centre (6.35, 17.78) radius 0.3574
  circle A201 centre (8.89, 17.78) radius 0.3574
  circle A202 centre (3.81, 30.48) radius 0.6033
  line L435 (32.077, 31.134) -> (32.077, 29.8767)
  line L436 (32.077, 29.8767) -> (32.077, 29.826)
  circle A203 centre (34.29, 30.48) radius 0.47
  circle A204 centre (31.75, 30.48) radius 0.47
  circle A205 centre (29.21, 30.48) radius 0.47
  circle A206 centre (26.67, 30.48) radius 0.47
  circle A207 centre (24.13, 30.48) radius 0.47
  circle A208 centre (21.59, 30.48) radius 0.47
  circle A209 centre (19.05, 30.48) radius 0.47
  circle A210 centre (16.51, 30.48) radius 0.47
  circle A211 centre (34.29, 17.78) radius 0.47
  circle A212 centre (31.75, 17.78) radius 0.47
  circle A213 centre (29.21, 17.78) radius 0.47
  circle A214 centre (26.67, 17.78) radius 0.47
  circle A215 centre (24.13, 17.78) radius 0.47
  circle A216 centre (21.59, 17.78) radius 0.47
  circle A217 centre (19.05, 17.78) radius 0.47
  circle A218 centre (16.51, 17.78) radius 0.47
  line L437 (34.29, 29.8926) -> (34.29, 30.01)
  line L438 (34.29, 29.8926) -> (34.29, 30.01)
  line L439 (33.963, 30.0736) -> (33.963, 30.1424)
  point P0 (15.24, 14.478)
  point P1 (33.02, 7.62)
  point P2 (24.13, 25.4)
  point P3 (7.62, 12.7)
  point P4 (7.62, 7.62)
  point P5 (7.62, 17.78)
  point P6 (3.683, 11.43)
  point P7 (36.83, 11.43)
  point P8 (7.62, 2.54)
  point P9 (17.78, 8.89)
  point P10 (19.05, 11.811)
  dimension "d2" = 0.94
  dimension "d5" = 0.94
  dimension "d8" = 2.54
  dimension "d13" = 0.94
  dimension "d16" = 2.54
  constraints: 880 end point, 335 point on circle, 205 centre point, 14 coincident, 10 concentric, 3 horizontal, 3 point on line, 2 parallel, 1 midpoint, 1 perpendicular, 1 tangent, 1 vertical, 70 other
  measures "d2" diameter of A173
  measures "d5" diameter of A203
  measures "d8" distance of A203.centre A204.centre
  measures "d13" diameter of A211
  measures "d16" distance of A211.centre A212.centre
extrude "Выдавливание3" add sketch "Эскиз1" along normal blind 2 contours L6 L5 L4 L3 A29 L8 A16 A12 L9 A15 A13 L7 A19 | A19 L7 L3 | L7 L9 L8 L3 A17 L15 A21 A28 L14 A23 A20 L12 A10 | A13 A15 L9 L7 | A10 L12 L3 | L3 L8 A29 | L12 A18 L3 | L12 L14 L15 A27 L3 A18 | A20 A23 L14 L12 | A12 A16 L8 L9 | A27 L15 L3 | L3 L15 A17 | L15 L14 A28 A21 | L20 L19 L18 L17 | L28 L27 L26 L25 | L36 L35 L34 L33 | A75 A74 | A79 A78 | L41 L42 L43 L44 L45 L46 L47 L48 | A147 A146 | A151 A150 | A155 A154 | A159 A158 | A163 A162 | A167 A166
